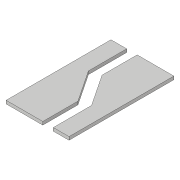
# Autodesk Inventor part: wall_2
Saved by Autodesk Inventor 2019 (Build 230136000, 136)
## iProperties
Created: 2021-05-31
Part Number: wall_2
Material: Generic
Document SubType Name: Modeling
Designer: dmulr
Density: 1 g/cm^3
Appearance: Default
Author: dmulr
Autodesk Inventor part; units mm, degrees
ref_plane "YZ Plane" through (0, 0, 0) normal (1, 0, 0) x (0, 1, 0)
ref_plane "XZ Plane" through (0, 0, 0) normal (0, 1, 0) x (-1, 0, 0)
ref_plane "XY Plane" through (0, 0, 0) normal (0, 0, 1) x (1, 0, 0)
sketch "Sketch1" plane through (0, 0, 0) normal (0, 1, 0) x (-1, 0, 0)
  line L0 (6000, 0) -> (6000, -10000)
  line L1 (0, -10000) -> (0, 0)
  line L2 (2000, 0) -> (2000, -10000) construction
  line L3 (4000, -10000) -> (4000, 0) construction
  line L4 (1500, 0) -> (1500, -3651.3878)
  line L5 (4500, -10000) -> (4500, -6348.6122)
  line L6 (2000, -3500) -> (4000, -6500) construction
  line L7 (2500, -3348.6122) -> (4500, -6348.6122)
  line L8 (1500, -3651.3878) -> (3500, -6651.3878)
  line L9 (2500, 0) -> (2500, -3348.6122)
  line L10 (3500, -10000) -> (3500, -6651.3878)
  line L11 (0, 0) -> (1500, 0)
  line L12 (2500, 0) -> (6000, 0)
  line L13 (6000, -10000) -> (4500, -10000)
  line L14 (3500, -10000) -> (0, -10000)
  dimension "d0" = 6000
  dimension "d1" = 10000
  dimension "d2" = 2000
  dimension "d3" = 2000
  dimension "d4" = 1000
  dimension "d10" = 500
  dimension "d11" = 500
  constraints: 30 end point, 11 parallel, 6 perpendicular, 4 point on line, 2 horizontal
  measures "d0" distance of L1.end L0.start
  measures "d1" distance of L1.start L1.end
  measures "d2" distance between parallel lines of L1 L2
  measures "d3" distance between parallel lines of L3 L0
  measures "d4" distance of L4.start L9.start
  measures "d10" distance between parallel lines of L6 L7
  measures "d11" distance between parallel lines of L8 L6
extrude "Extrusion1" add sketch "Sketch1" along normal blind 300
body "Solid1"
